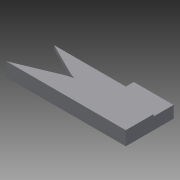
# Autodesk Inventor part: clip_tip_M
Saved by Autodesk Inventor 2015 (Build 190159000, 159)
## iProperties
Created: 2017-10-02
Part Number: clip_tip_M
Material: Generic
Document SubType Name: Modeling
Designer: Anshul
Density: 1 g/cm^3
Appearance: Default
Author: Anshul
Autodesk Inventor part; units mm, degrees
ref_plane "YZ Plane" through (0, 0, 0) normal (1, 0, 0) x (0, 1, 0)
ref_plane "XZ Plane" through (0, 0, 0) normal (0, 1, 0) x (-1, 0, 0)
ref_plane "XY Plane" through (0, 0, 0) normal (0, 0, 1) x (1, 0, 0)
sketch "Sketch1" plane through (0, 0, 0) normal (0, 1, 0) x (-1, 0, 0)
  line L0 (0, 0) -> (30, 0)
  line L1 (0, 5) -> (0, 0)
  line L2 (20, 5) -> (30, 0)
  line L3 (30, 12) -> (0, 12)
  line L4 (0, 12) -> (0, 5)
  line L5 (0, 5) -> (0, 7)
  line L6 (18, 7) -> (30, 12)
  line L7 (20, 5) -> (10, 5)
  line L8 (10, 5) -> (10, 7)
  line L9 (18, 7) -> (10, 7)
  line L10 (10, 5) -> (0, 5)
  line L11 (10, 5) -> (10, 0)
  dimension "d13" = 2
  dimension "d15" = 10
  constraints: 24 end point, 3 perpendicular, 3 point on line, 2 horizontal
  measures "d13" distance of L1.start L5.end
  measures "d15" distance of L2.start L7.end
extrude "Extrusion6" add sketch "Sketch1" along normal blind 1 contours L11 L7 L2 L0
extrude "Extrusion7" add sketch "Sketch1" along normal blind 3 contours L1 L10 L11 L0
extrude "Extrusion8" add sketch "Sketch1" along normal blind 3.5 contours L4 L3 L6 L9 L8 L10
fillet "Fillet4" radius 10 2 edges at (-20, 0.5, 5) (-18, 1.75, 7)
body "Solid2"
